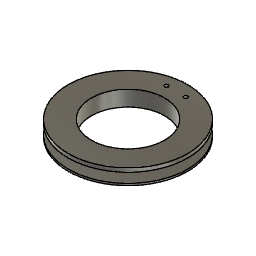
Coil v11 (Autodesk Fusion 360 design; units mm, degrees)
Autodesk Fusion 360 part; units mm, degrees
note: some values were not read from the file. Set by a fixed rule: which sketch regions a step uses.
sketch "Sketch1" plane through (0, 0, 0) normal (0, 0, 1) x (1, 0, 0)
  circle A0 centre (0, 0) radius 9.5
  circle A1 centre (0, 0) radius 10.5
  circle A2 centre (0, 0) radius 15.5
  dimension "d1" = 19
  dimension "d2" = 1
  dimension "d3" = 6
  constraint coincident A0.centre A1.centre
  measures "d1" diameter of A0
extrude "Extrude2" add sketch "Sketch1" along normal blind 0.5 contours A2 makes body 1
extrude "Extrude1" add sketch "Sketch1" along normal blind 3 separate body contours A1 makes body 2
sketch "Sketch2" plane through (0, 0, 3) normal (0, 0, 1) x (-1, 0, 0)
  circle A0 centre (0, 0) radius 9.5
  circle A1 centre (0, 0) radius 10.5
  circle A2 centre (0, 0) radius 15.5
  dimension "d8" = 31
  constraint coincident A0.centre A1.centre
  measures "d8" diameter of A2
extrude "Extrude3" add sketch "Sketch2" along normal blind 1 contours A1 | A2 bodies 2
sketch "Sketch4" plane through (0, 0, 4) normal (0, 0, 1) x (-1, 0, 0)
  circle A0 centre (0, 0) radius 9.5
  circle A1 centre (0, 0) radius 15.5
  line L0 (0, 0) -> (0, -15.5) construction
  line L1 (0, -9.5) -> (0, -15.5) construction
  line L2 (0, -12.5) -> (9.1652, -12.5) construction
  line L3 (9.1652, -12.5) -> (0, -12.5) construction
  line L4 (-9.1652, -12.5) -> (0, -12.5) construction
  line L5 (0, -12.5) -> (2.5, -12.5) construction
  line L6 (0, -12.5) -> (-2.5, -12.5) construction
  circle A2 centre (2.5, -12.5) radius 0.5
  circle A3 centre (-2.5, -12.5) radius 0.5
  dimension "d25" = 2.5
  dimension "d26" = 2.5
  dimension "d27" = 1
  dimension "d28" = 1
  constraint coincident A0.centre A1.centre
  constraint coincident A1 L0.end
  constraint vertical L0
  constraint coincident L0 L1.start
  constraint coincident A0 L1.start
  constraint midpoint L1 L2.start
  constraint coincident A1 L2.end
  constraint perpendicular L0 L2
  constraint coincident A1 L4.start
  constraint perpendicular L1 L4
  constraint perpendicular L1 L5
  constraint perpendicular L0 L6
  constraint coincident L5.end A2.centre
  constraint coincident L6.end A3.centre
  measures "d25" distance of L2.start L5.end
  measures "d26" distance of L2.start L6.end
  measures "d27" diameter of A2
  measures "d28" diameter of A3
sketch "Sketch9" plane through (0, 0, 0) normal (0, 1, 0) x (1, 0, 0)
  line L0 (18.5, -6) -> (16.534, -6) construction
  line L1 (16.534, -6) -> (18.5, -6) construction
  line L2 (10.5, -1) -> (10.5, -3)
  line L3 (10.5, -3) -> (10.5, -2)
  line L4 (15.5, -3) -> (10.5, -3)
  line L5 (10.5, -1) -> (15.5, -3)
  constraint vertical L2
  constraint midpoint L2 L3.end
revolve "Revolve1" add sketch "Sketch9" angle 360 about axis through (0, 0, 1.75) along (0, 0, 1) bodies 2
extrude "Extrude5" cut sketch "Sketch4" against normal blind 3 contours A2 | A3 bodies 2
combine "Combine1" operation add target body 2 tool bodies 1
